Autodesk Fusion 360 part; units mm, degrees
note: some values were not read from the file. Chosen so that the rebuilt part matches the saved one: which face or edge a step refers to.
(part 2 of 2)
  spline S171 degree 3 poles (-22.5654, 6.7875) (-22.5201, 6.8696) (-22.457, 6.9326) (-22.3762, 6.9767) knots 0 0 0 0 1 1 1 1
  spline S172 degree 3 poles (-22.3762, 6.9767) (-22.2941, 7.022) (-22.2081, 7.045) (-22.1187, 7.045) knots 0 0 0 0 1 1 1 1
extrude "Extrude5" add sketch "Sketch5" along normal blind 2 contours L4 S0 S1 L5 S2 S3 L6 S4 S5 L7 S6 S7 | S8 L8 L9 S9 S10 L10 S11 L11 S12 | L12 S13 S14 L13 L14 L15 S15 S16 L16 S17 L17 S18 | S19 L18 S20 S21 L19 S22 | S23 S24 S25 S26 S27 S28 S29 L20 L21 S30 S31 L22 L23 S32 S33 S34 | L24 S35 S36 L25 L26 S37 S38 L27 L28 S39 S40 | S41 S42 S43 S44 S45 S46 S47 S48 S49 S50 S51 S52 S53 S54 L29 | S55 S56 L33 S57 L34 S58 S59 L35 S60 S61 L36 S62 L37 S63 S64 L38 | S65 S66 S67 S68 S69 S70 S71 S72 S73 S74 S75 S76 | S89 S90 S91 S92 S93 S94 S95 S96 S97 S98 S99 S100 | S101 S102 S103 S104 S105 S106 S107 S108 S109 S110 S111 S112 | S125 S126 S127 S128 S129 S130 S131 S132 S133 S134 S135 S136 | S137 S138 S139 S140 S141 S142 S143 S144 S145 S146 S147 S148 | S161 S162 S163 S164 S165 S166 S167 S168 S169 S170 S171 S172
extrude "Extrude2" [suppressed]
sketch "Sketch3" plane through (0, 0, 0) normal (1, 0, 0) x (0, 1, 0)
  line L0 (-62.5649, -7.7043) -> (-61.5927, -7.7068)
  spline S0 degree 3 poles (-61.5927, -7.7068) (-61.2707, -7.7117) (-61.1085, -7.8721) (-61.1066, -8.188) knots 0 0 0 0 1 1 1 1
  spline S1 degree 3 poles (-61.1066, -8.188) (-61.1085, -8.5155) (-61.2713, -8.6784) (-61.5952, -8.6765) knots 0 0 0 0 1 1 1 1
  line L1 (-61.5952, -8.6765) -> (-62.5625, -8.679)
  spline S2 degree 3 poles (-62.5625, -8.679) (-63.2089, -8.6741) (-63.5322, -8.9967) (-63.5322, -9.6462) knots 0 0 0 0 1 1 1 1
  spline S3 degree 3 poles (-63.5322, -9.6462) (-63.5322, -10.2915) (-63.2089, -10.6154) (-62.5625, -10.6184) knots 0 0 0 0 1 1 1 1
  line L2 (-62.5625, -10.6184) -> (-61.5952, -10.6184)
  spline S4 degree 3 poles (-61.5952, -10.6184) (-61.2713, -10.6252) (-61.1091, -10.7856) (-61.1091, -11.0996) knots 0 0 0 0 1 1 1 1
  spline S5 degree 3 poles (-61.1091, -11.0996) (-61.1091, -11.4241) (-61.2695, -11.5869) (-61.5903, -11.5882) knots 0 0 0 0 1 1 1 1
  line L3 (-61.5903, -11.5882) -> (-62.5625, -11.5882)
  spline S6 degree 3 poles (-62.5625, -11.5882) (-63.8573, -11.5882) (-64.5056, -10.9404) (-64.5068, -9.6438) knots 0 0 0 0 1 1 1 1
  spline S7 degree 3 poles (-64.5068, -9.6438) (-64.5068, -8.3496) (-63.8597, -7.7031) (-62.5649, -7.7043) knots 0 0 0 0 1 1 1 1
  spline S8 degree 3 poles (-60.1369, -7.6994) (-59.8112, -7.708) (-59.6471, -7.8666) (-59.6434, -8.1756) knots 0 0 0 0 1 1 1 1
  line L4 (-59.6434, -8.1756) -> (-59.6483, -10.6135)
  line L5 (-59.6483, -10.6135) -> (-57.7187, -10.6135)
  spline S9 degree 3 poles (-57.7187, -10.6135) (-57.3918, -10.6154) (-57.2277, -10.7788) (-57.2277, -11.1045) knots 0 0 0 0 1 1 1 1
  spline S10 degree 3 poles (-57.2277, -11.1045) (-57.2296, -11.4241) (-57.3899, -11.5851) (-57.7089, -11.5882) knots 0 0 0 0 1 1 1 1
  line L6 (-57.7089, -11.5882) -> (-60.1369, -11.5882)
  spline S11 degree 3 poles (-60.1369, -11.5882) (-60.4595, -11.5882) (-60.6217, -11.4315) (-60.623, -11.1169) knots 0 0 0 0 1 1 1 1
  line L7 (-60.623, -11.1169) -> (-60.623, -8.1904)
  spline S12 degree 3 poles (-60.623, -8.1904) (-60.6217, -7.8697) (-60.4595, -7.7062) (-60.1369, -7.6994) knots 0 0 0 0 1 1 1 1
  line L8 (-56.253, -7.6994) -> (-53.7954, -7.7043)
  spline S13 degree 3 poles (-53.7954, -7.7043) (-53.4931, -7.7093) (-53.3408, -7.8666) (-53.3389, -8.1756) knots 0 0 0 0 1 1 1 1
  spline S14 degree 3 poles (-53.3389, -8.1756) (-53.3389, -8.5063) (-53.503, -8.6741) (-53.8299, -8.679) knots 0 0 0 0 1 1 1 1
  line L9 (-53.8299, -8.679) -> (-55.7644, -8.679)
  line L10 (-55.7644, -8.679) -> (-55.7644, -10.6135)
  line L11 (-55.7644, -10.6135) -> (-53.8349, -10.6135)
  spline S15 degree 3 poles (-53.8349, -10.6135) (-53.5079, -10.6154) (-53.3438, -10.7788) (-53.3438, -11.1045) knots 0 0 0 0 1 1 1 1
  spline S16 degree 3 poles (-53.3438, -11.1045) (-53.3457, -11.4241) (-53.5061, -11.5851) (-53.825, -11.5882) knots 0 0 0 0 1 1 1 1
  line L12 (-53.825, -11.5882) -> (-56.253, -11.5882)
  spline S17 degree 3 poles (-56.253, -11.5882) (-56.5756, -11.5882) (-56.7379, -11.4315) (-56.7391, -11.1169) knots 0 0 0 0 1 1 1 1
  line L13 (-56.7391, -11.1169) -> (-56.7391, -8.1904)
  spline S18 degree 3 poles (-56.7391, -8.1904) (-56.7379, -7.8697) (-56.5756, -7.7062) (-56.253, -7.6994) knots 0 0 0 0 1 1 1 1
  spline S19 degree 3 poles (-55.5325, -9.6561) (-55.5294, -9.3341) (-55.369, -9.17) (-55.0513, -9.1651) knots 0 0 0 0 1 1 1 1
  line L14 (-55.0513, -9.1651) -> (-54.0742, -9.1651)
  spline S20 degree 3 poles (-54.0742, -9.1651) (-53.7504, -9.1688) (-53.5857, -9.3304) (-53.5807, -9.6512) knots 0 0 0 0 1 1 1 1
  spline S21 degree 3 poles (-53.5807, -9.6512) (-53.5875, -9.9757) (-53.751, -10.1373) (-54.0718, -10.1373) knots 0 0 0 0 1 1 1 1
  line L15 (-54.0718, -10.1373) -> (-55.0489, -10.1373)
  spline S22 degree 3 poles (-55.0489, -10.1373) (-55.3696, -10.1391) (-55.5313, -9.9787) (-55.5325, -9.6561) knots 0 0 0 0 1 1 1 1
  spline S23 degree 3 poles (-52.3617, -7.6945) (-52.2007, -7.6945) (-52.0792, -7.7352) (-51.9966, -7.8154) knots 0 0 0 0 1 1 1 1
  spline S24 degree 3 poles (-51.9966, -7.8154) (-51.9145, -7.8943) (-51.6264, -8.2324) (-51.1329, -8.8295) knots 0 0 0 0 1 1 1 1
  spline S25 degree 3 poles (-51.1329, -8.8295) (-50.6314, -8.2225) (-50.3396, -7.8795) (-50.257, -7.8006) knots 0 0 0 0 1 1 1 1
  spline S26 degree 3 poles (-50.257, -7.8006) (-50.1749, -7.7216) (-50.0534, -7.6821) (-49.8918, -7.6821) knots 0 0 0 0 1 1 1 1
  spline S27 degree 3 poles (-49.8918, -7.6821) (-49.7339, -7.6821) (-49.6123, -7.7235) (-49.5266, -7.8055) knots 0 0 0 0 1 1 1 1
  spline S28 degree 3 poles (-49.5266, -7.8055) (-49.4415, -7.8882) (-49.4008, -8.0103) (-49.4057, -8.1732) knots 0 0 0 0 1 1 1 1
  spline S29 degree 3 poles (-49.4057, -8.1732) (-49.4057, -8.3446) (-49.4914, -8.505) (-49.6623, -8.6543) knots 0 0 0 0 1 1 1 1
  line L16 (-49.6623, -8.6543) -> (-50.6567, -9.814)
  line L17 (-50.6567, -9.814) -> (-50.6592, -11.1045)
  spline S30 degree 3 poles (-50.6592, -11.1045) (-50.666, -11.4222) (-50.8288, -11.5832) (-51.1477, -11.5882) knots 0 0 0 0 1 1 1 1
  spline S31 degree 3 poles (-51.1477, -11.5882) (-51.4685, -11.5962) (-51.6289, -11.4302) (-51.6289, -11.0897) knots 0 0 0 0 1 1 1 1
  line L18 (-51.6289, -11.0897) -> (-51.6338, -9.8091)
  line L19 (-51.6338, -9.8091) -> (-52.5912, -8.6691)
  spline S32 degree 3 poles (-52.5912, -8.6691) (-52.7627, -8.518) (-52.8478, -8.357) (-52.8478, -8.1855) knots 0 0 0 0 1 1 1 1
  spline S33 degree 3 poles (-52.8478, -8.1855) (-52.8528, -8.0214) (-52.8133, -7.8986) (-52.7294, -7.8178) knots 0 0 0 0 1 1 1 1
  spline S34 degree 3 poles (-52.7294, -7.8178) (-52.6443, -7.7358) (-52.5215, -7.6945) (-52.3617, -7.6945) knots 0 0 0 0 1 1 1 1
  line L20 (-48.4804, -7.6994) -> (-46.0228, -7.7043)
  spline S35 degree 3 poles (-46.0228, -7.7043) (-45.7205, -7.7093) (-45.5682, -7.8666) (-45.5663, -8.1756) knots 0 0 0 0 1 1 1 1
  spline S36 degree 3 poles (-45.5663, -8.1756) (-45.5663, -8.5063) (-45.7304, -8.6741) (-46.0574, -8.679) knots 0 0 0 0 1 1 1 1
  line L21 (-46.0574, -8.679) -> (-46.7828, -8.679)
  line L22 (-46.7828, -8.679) -> (-46.7803, -11.1045)
  spline S37 degree 3 poles (-46.7803, -11.1045) (-46.784, -11.4241) (-46.9469, -11.5851) (-47.2689, -11.5882) knots 0 0 0 0 1 1 1 1
  spline S38 degree 3 poles (-47.2689, -11.5882) (-47.5934, -11.5882) (-47.755, -11.4315) (-47.755, -11.1169) knots 0 0 0 0 1 1 1 1
  line L23 (-47.755, -11.1169) -> (-47.7525, -8.679)
  line L24 (-47.7525, -8.679) -> (-48.4804, -8.679)
  spline S39 degree 3 poles (-48.4804, -8.679) (-48.8049, -8.679) (-48.9665, -8.5161) (-48.9665, -8.1904) knots 0 0 0 0 1 1 1 1
  spline S40 degree 3 poles (-48.9665, -8.1904) (-48.9653, -7.8697) (-48.803, -7.7062) (-48.4804, -7.6994) knots 0 0 0 0 1 1 1 1
  spline S41 degree 3 poles (-44.5941, -11.5906) (-44.6768, -11.5906) (-44.7563, -11.5703) (-44.8334, -11.5289) knots 0 0 0 0 1 1 1 1
  spline S42 degree 3 poles (-44.8334, -11.5289) (-44.9112, -11.4882) (-44.9716, -11.429) (-45.016, -11.3513) knots 0 0 0 0 1 1 1 1
  spline S43 degree 3 poles (-45.016, -11.3513) (-45.0592, -11.2723) (-45.0802, -11.1903) (-45.0802, -11.1045) knots 0 0 0 0 1 1 1 1
  spline S44 degree 3 poles (-45.0802, -11.1045) (-45.0802, -11.0206) (-44.8384, -10.4926) (-44.3547, -9.5204) knots 0 0 0 0 1 1 1 1
  spline S45 degree 3 poles (-44.3547, -9.5204) (-43.8699, -8.547) (-43.6065, -8.0214) (-43.5652, -7.9437) knots 0 0 0 0 1 1 1 1
  spline S46 degree 3 poles (-43.5652, -7.9437) (-43.5226, -7.8666) (-43.4628, -7.8067) (-43.385, -7.7636) knots 0 0 0 0 1 1 1 1
  spline S47 degree 3 poles (-43.385, -7.7636) (-43.3079, -7.721) (-43.2265, -7.6994) (-43.1407, -7.6994) knots 0 0 0 0 1 1 1 1
  spline S48 degree 3 poles (-43.1407, -7.6994) (-43.0569, -7.6994) (-42.9773, -7.721) (-42.9014, -7.7636) knots 0 0 0 0 1 1 1 1
  spline S49 degree 3 poles (-42.9014, -7.7636) (-42.8243, -7.8067) (-42.7645, -7.8666) (-42.7213, -7.9437) knots 0 0 0 0 1 1 1 1
  spline S50 degree 3 poles (-42.7213, -7.9437) (-42.6787, -8.0214) (-42.4141, -8.547) (-41.9267, -9.5204) knots 0 0 0 0 1 1 1 1
  spline S51 degree 3 poles (-41.9267, -9.5204) (-41.44, -10.4926) (-41.1964, -11.0206) (-41.1964, -11.1045) knots 0 0 0 0 1 1 1 1
  spline S52 degree 3 poles (-41.1964, -11.1045) (-41.1964, -11.1903) (-41.2186, -11.2723) (-41.263, -11.3513) knots 0 0 0 0 1 1 1 1
  spline S53 degree 3 poles (-41.263, -11.3513) (-41.3062, -11.429) (-41.3666, -11.4882) (-41.4456, -11.5289) knots 0 0 0 0 1 1 1 1
  spline S54 degree 3 poles (-41.4456, -11.5289) (-41.5233, -11.5703) (-41.6023, -11.5906) (-41.6825, -11.5906) knots 0 0 0 0 1 1 1 1
  line L25 (-41.6825, -11.5906) -> (-44.5941, -11.5906)
  line L26 (-42.477, -10.611) -> (-43.1407, -9.244)
  line L27 (-43.1407, -9.244) -> (-43.8094, -10.611)
  line L28 (-43.8094, -10.611) -> (-42.477, -10.611)
  spline S55 degree 3 poles (-36.5839, -7.7043) (-35.4507, -7.7031) (-34.8832, -8.3502) (-34.8814, -9.6462) knots 0 0 0 0 1 1 1 1
  spline S56 degree 3 poles (-34.8814, -9.6462) (-34.8801, -9.9707) (-35.0418, -10.1317) (-35.3675, -10.1299) knots 0 0 0 0 1 1 1 1
  line L29 (-35.3675, -10.1299) -> (-37.3118, -10.1274)
  spline S57 degree 3 poles (-37.3118, -10.1274) (-37.3088, -10.4531) (-37.0669, -10.6172) (-36.5864, -10.6184) knots 0 0 0 0 1 1 1 1
  line L30 (-36.5864, -10.6184) -> (-35.365, -10.6135)
  spline S58 degree 3 poles (-35.365, -10.6135) (-35.0479, -10.6154) (-34.8863, -10.7782) (-34.8814, -11.1021) knots 0 0 0 0 1 1 1 1
  spline S59 degree 3 poles (-34.8814, -11.1021) (-34.8832, -11.4278) (-35.0455, -11.5894) (-35.3675, -11.5882) knots 0 0 0 0 1 1 1 1
  line L31 (-35.3675, -11.5882) -> (-36.579, -11.5882)
  spline S60 degree 3 poles (-36.579, -11.5882) (-37.7159, -11.5869) (-38.2853, -10.9386) (-38.2865, -9.6438) knots 0 0 0 0 1 1 1 1
  spline S61 degree 3 poles (-38.2865, -9.6438) (-38.2853, -9.323) (-38.123, -9.162) (-37.8004, -9.1602) knots 0 0 0 0 1 1 1 1
  line L32 (-37.8004, -9.1602) -> (-35.856, -9.1626)
  spline S62 degree 3 poles (-35.856, -9.1626) (-35.856, -8.8388) (-36.0954, -8.6778) (-36.5741, -8.679) knots 0 0 0 0 1 1 1 1
  line L33 (-36.5741, -8.679) -> (-37.7955, -8.679)
  spline S63 degree 3 poles (-37.7955, -8.679) (-38.1162, -8.671) (-38.2803, -8.5075) (-38.2865, -8.188) knots 0 0 0 0 1 1 1 1
  spline S64 degree 3 poles (-38.2865, -8.188) (-38.2785, -7.8641) (-38.115, -7.7031) (-37.7955, -7.7043) knots 0 0 0 0 1 1 1 1
  line L34 (-37.7955, -7.7043) -> (-36.5839, -7.7043)
  spline S65 degree 3 poles (-32.4583, -7.7043) (-32.1326, -7.7043) (-31.8155, -7.7882) (-31.5058, -7.956) knots 0 0 0 0 1 1 1 1
  spline S66 degree 3 poles (-31.5058, -7.956) (-31.1949, -8.1238) (-30.9519, -8.3644) (-30.7755, -8.6765) knots 0 0 0 0 1 1 1 1
  spline S67 degree 3 poles (-30.7755, -8.6765) (-30.5997, -8.9874) (-30.5115, -9.3119) (-30.5115, -9.6487) knots 0 0 0 0 1 1 1 1
  spline S68 degree 3 poles (-30.5115, -9.6487) (-30.5115, -9.9861) (-30.5972, -10.3094) (-30.7681, -10.6184) knots 0 0 0 0 1 1 1 1
  spline S69 degree 3 poles (-30.7681, -10.6184) (-30.9396, -10.9263) (-31.1795, -11.1656) (-31.4886, -11.3365) knots 0 0 0 0 1 1 1 1
  spline S70 degree 3 poles (-31.4886, -11.3365) (-31.7982, -11.508) (-32.1215, -11.5931) (-32.4583, -11.5931) knots 0 0 0 0 1 1 1 1
  spline S71 degree 3 poles (-32.4583, -11.5931) (-32.7939, -11.5931) (-33.1165, -11.508) (-33.4256, -11.3365) knots 0 0 0 0 1 1 1 1
  spline S72 degree 3 poles (-33.4256, -11.3365) (-33.7352, -11.1656) (-33.9752, -10.9263) (-34.1461, -10.6184) knots 0 0 0 0 1 1 1 1
  spline S73 degree 3 poles (-34.1461, -10.6184) (-34.3176, -10.3094) (-34.4027, -9.9861) (-34.4027, -9.6487) knots 0 0 0 0 1 1 1 1
  spline S74 degree 3 poles (-34.4027, -9.6487) (-34.4027, -9.3119) (-34.3163, -8.9874) (-34.1436, -8.6765) knots 0 0 0 0 1 1 1 1
  spline S75 degree 3 poles (-34.1436, -8.6765) (-33.9696, -8.3644) (-33.7278, -8.1238) (-33.4182, -7.956) knots 0 0 0 0 1 1 1 1
  spline S76 degree 3 poles (-33.4182, -7.956) (-33.1072, -7.7882) (-32.7877, -7.7043) (-32.4583, -7.7043) knots 0 0 0 0 1 1 1 1
  spline S77 degree 3 poles (-32.4558, -8.6716) (-32.6205, -8.6716) (-32.7803, -8.7135) (-32.9345, -8.7974) knots 0 0 0 0 1 1 1 1
  spline S78 degree 3 poles (-32.9345, -8.7974) (-33.0894, -8.8801) (-33.2103, -8.9991) (-33.2972, -9.1552) knots 0 0 0 0 1 1 1 1
  spline S79 degree 3 poles (-33.2972, -9.1552) (-33.3848, -9.3119) (-33.428, -9.4748) (-33.428, -9.6438) knots 0 0 0 0 1 1 1 1
  spline S80 degree 3 poles (-33.428, -9.6438) (-33.428, -9.8134) (-33.3855, -9.9757) (-33.2997, -10.1299) knots 0 0 0 0 1 1 1 1
  spline S81 degree 3 poles (-33.2997, -10.1299) (-33.2146, -10.2829) (-33.0943, -10.4025) (-32.9395, -10.4877) knots 0 0 0 0 1 1 1 1
  spline S82 degree 3 poles (-32.9395, -10.4877) (-32.7852, -10.5734) (-32.6236, -10.616) (-32.4558, -10.616) knots 0 0 0 0 1 1 1 1
  spline S83 degree 3 poles (-32.4558, -10.616) (-32.2868, -10.616) (-32.1246, -10.5734) (-31.9697, -10.4877) knots 0 0 0 0 1 1 1 1
  spline S84 degree 3 poles (-31.9697, -10.4877) (-31.8155, -10.4025) (-31.6952, -10.2829) (-31.6095, -10.1299) knots 0 0 0 0 1 1 1 1
  spline S85 degree 3 poles (-31.6095, -10.1299) (-31.5244, -9.9757) (-31.4812, -9.8134) (-31.4812, -9.6438) knots 0 0 0 0 1 1 1 1
  spline S86 degree 3 poles (-31.4812, -9.6438) (-31.4812, -9.4748) (-31.525, -9.3119) (-31.612, -9.1552) knots 0 0 0 0 1 1 1 1
  spline S87 degree 3 poles (-31.612, -9.1552) (-31.6995, -8.9991) (-31.8211, -8.8801) (-31.9771, -8.7974) knots 0 0 0 0 1 1 1 1
  spline S88 degree 3 poles (-31.9771, -8.7974) (-32.132, -8.7135) (-32.2917, -8.6716) (-32.4558, -8.6716) knots 0 0 0 0 1 1 1 1
  spline S89 degree 3 poles (-32.4583, -9.17) (-32.3781, -9.17) (-32.2998, -9.1916) (-32.2239, -9.2342) knots 0 0 0 0 1 1 1 1
  spline S90 degree 3 poles (-32.2239, -9.2342) (-32.1468, -9.2755) (-32.0869, -9.3347) (-32.0438, -9.4118) knots 0 0 0 0 1 1 1 1
  spline S91 degree 3 poles (-32.0438, -9.4118) (-31.9993, -9.4877) (-31.9771, -9.5685) (-31.9771, -9.6536) knots 0 0 0 0 1 1 1 1
  spline S92 degree 3 poles (-31.9771, -9.6536) (-31.9771, -9.7375) (-31.9987, -9.8184) (-32.0413, -9.8955) knots 0 0 0 0 1 1 1 1
  spline S93 degree 3 poles (-32.0413, -9.8955) (-32.0845, -9.9713) (-32.1437, -10.0306) (-32.219, -10.0731) knots 0 0 0 0 1 1 1 1
  spline S94 degree 3 poles (-32.219, -10.0731) (-32.2948, -10.1145) (-32.3744, -10.1348) (-32.4583, -10.1348) knots 0 0 0 0 1 1 1 1
  spline S95 degree 3 poles (-32.4583, -10.1348) (-32.544, -10.1348) (-32.6255, -10.1145) (-32.7026, -10.0731) knots 0 0 0 0 1 1 1 1
  spline S96 degree 3 poles (-32.7026, -10.0731) (-32.7785, -10.0306) (-32.8377, -9.9713) (-32.8802, -9.8955) knots 0 0 0 0 1 1 1 1
  spline S97 degree 3 poles (-32.8802, -9.8955) (-32.9216, -9.8184) (-32.9419, -9.7375) (-32.9419, -9.6536) knots 0 0 0 0 1 1 1 1
  spline S98 degree 3 poles (-32.9419, -9.6536) (-32.9419, -9.5685) (-32.921, -9.4877) (-32.8778, -9.4118) knots 0 0 0 0 1 1 1 1
  spline S99 degree 3 poles (-32.8778, -9.4118) (-32.8352, -9.3347) (-32.776, -9.2755) (-32.7001, -9.2342) knots 0 0 0 0 1 1 1 1
  spline S100 degree 3 poles (-32.7001, -9.2342) (-32.623, -9.1916) (-32.5422, -9.17) (-32.4583, -9.17) knots 0 0 0 0 1 1 1 1
  spline S101 degree 3 poles (-28.0838, -7.7043) (-27.7581, -7.7043) (-27.441, -7.7882) (-27.1313, -7.956) knots 0 0 0 0 1 1 1 1
  spline S102 degree 3 poles (-27.1313, -7.956) (-26.8204, -8.1238) (-26.5774, -8.3644) (-26.401, -8.6765) knots 0 0 0 0 1 1 1 1
  spline S103 degree 3 poles (-26.401, -8.6765) (-26.2252, -8.9874) (-26.1369, -9.3119) (-26.1369, -9.6487) knots 0 0 0 0 1 1 1 1
  spline S104 degree 3 poles (-26.1369, -9.6487) (-26.1369, -9.9861) (-26.2227, -10.3094) (-26.3936, -10.6184) knots 0 0 0 0 1 1 1 1
  spline S105 degree 3 poles (-26.3936, -10.6184) (-26.5651, -10.9263) (-26.805, -11.1656) (-27.1141, -11.3365) knots 0 0 0 0 1 1 1 1
  spline S106 degree 3 poles (-27.1141, -11.3365) (-27.4237, -11.508) (-27.747, -11.5931) (-28.0838, -11.5931) knots 0 0 0 0 1 1 1 1
  spline S107 degree 3 poles (-28.0838, -11.5931) (-28.4194, -11.5931) (-28.742, -11.508) (-29.051, -11.3365) knots 0 0 0 0 1 1 1 1
  spline S108 degree 3 poles (-29.051, -11.3365) (-29.3607, -11.1656) (-29.6007, -10.9263) (-29.7716, -10.6184) knots 0 0 0 0 1 1 1 1
  spline S109 degree 3 poles (-29.7716, -10.6184) (-29.943, -10.3094) (-30.0282, -9.9861) (-30.0282, -9.6487) knots 0 0 0 0 1 1 1 1
  spline S110 degree 3 poles (-30.0282, -9.6487) (-30.0282, -9.3119) (-29.9418, -8.9874) (-29.7691, -8.6765) knots 0 0 0 0 1 1 1 1
  spline S111 degree 3 poles (-29.7691, -8.6765) (-29.5951, -8.3644) (-29.3533, -8.1238) (-29.0436, -7.956) knots 0 0 0 0 1 1 1 1
  spline S112 degree 3 poles (-29.0436, -7.956) (-28.7327, -7.7882) (-28.4132, -7.7043) (-28.0838, -7.7043) knots 0 0 0 0 1 1 1 1
  spline S113 degree 3 poles (-28.0813, -8.6716) (-28.246, -8.6716) (-28.4058, -8.7135) (-28.56, -8.7974) knots 0 0 0 0 1 1 1 1
  spline S114 degree 3 poles (-28.56, -8.7974) (-28.7149, -8.8801) (-28.8358, -8.9991) (-28.9227, -9.1552) knots 0 0 0 0 1 1 1 1
  spline S115 degree 3 poles (-28.9227, -9.1552) (-29.0103, -9.3119) (-29.0535, -9.4748) (-29.0535, -9.6438) knots 0 0 0 0 1 1 1 1
  spline S116 degree 3 poles (-29.0535, -9.6438) (-29.0535, -9.8134) (-29.0109, -9.9757) (-28.9252, -10.1299) knots 0 0 0 0 1 1 1 1
  spline S117 degree 3 poles (-28.9252, -10.1299) (-28.8401, -10.2829) (-28.7198, -10.4025) (-28.565, -10.4877) knots 0 0 0 0 1 1 1 1
  spline S118 degree 3 poles (-28.565, -10.4877) (-28.4107, -10.5734) (-28.2491, -10.616) (-28.0813, -10.616) knots 0 0 0 0 1 1 1 1
  spline S119 degree 3 poles (-28.0813, -10.616) (-27.9123, -10.616) (-27.7501, -10.5734) (-27.5952, -10.4877) knots 0 0 0 0 1 1 1 1
  spline S120 degree 3 poles (-27.5952, -10.4877) (-27.441, -10.4025) (-27.3207, -10.2829) (-27.235, -10.1299) knots 0 0 0 0 1 1 1 1
  spline S121 degree 3 poles (-27.235, -10.1299) (-27.1498, -9.9757) (-27.1067, -9.8134) (-27.1067, -9.6438) knots 0 0 0 0 1 1 1 1
  spline S122 degree 3 poles (-27.1067, -9.6438) (-27.1067, -9.4748) (-27.1505, -9.3119) (-27.2374, -9.1552) knots 0 0 0 0 1 1 1 1
  spline S123 degree 3 poles (-27.2374, -9.1552) (-27.325, -8.9991) (-27.4466, -8.8801) (-27.6026, -8.7974) knots 0 0 0 0 1 1 1 1
  spline S124 degree 3 poles (-27.6026, -8.7974) (-27.7575, -8.7135) (-27.9172, -8.6716) (-28.0813, -8.6716) knots 0 0 0 0 1 1 1 1
  spline S125 degree 3 poles (-28.0838, -9.17) (-28.0036, -9.17) (-27.9253, -9.1916) (-27.8494, -9.2342) knots 0 0 0 0 1 1 1 1
  spline S126 degree 3 poles (-27.8494, -9.2342) (-27.7723, -9.2755) (-27.7124, -9.3347) (-27.6693, -9.4118) knots 0 0 0 0 1 1 1 1
  spline S127 degree 3 poles (-27.6693, -9.4118) (-27.6248, -9.4877) (-27.6026, -9.5685) (-27.6026, -9.6536) knots 0 0 0 0 1 1 1 1
  spline S128 degree 3 poles (-27.6026, -9.6536) (-27.6026, -9.7375) (-27.6242, -9.8184) (-27.6668, -9.8955) knots 0 0 0 0 1 1 1 1
  spline S129 degree 3 poles (-27.6668, -9.8955) (-27.71, -9.9713) (-27.7692, -10.0306) (-27.8444, -10.0731) knots 0 0 0 0 1 1 1 1
  spline S130 degree 3 poles (-27.8444, -10.0731) (-27.9203, -10.1145) (-27.9999, -10.1348) (-28.0838, -10.1348) knots 0 0 0 0 1 1 1 1
  spline S131 degree 3 poles (-28.0838, -10.1348) (-28.1695, -10.1348) (-28.251, -10.1145) (-28.3281, -10.0731) knots 0 0 0 0 1 1 1 1
  spline S132 degree 3 poles (-28.3281, -10.0731) (-28.4039, -10.0306) (-28.4632, -9.9713) (-28.5057, -9.8955) knots 0 0 0 0 1 1 1 1
  spline S133 degree 3 poles (-28.5057, -9.8955) (-28.5471, -9.8184) (-28.5674, -9.7375) (-28.5674, -9.6536) knots 0 0 0 0 1 1 1 1
  spline S134 degree 3 poles (-28.5674, -9.6536) (-28.5674, -9.5685) (-28.5464, -9.4877) (-28.5033, -9.4118) knots 0 0 0 0 1 1 1 1
  spline S135 degree 3 poles (-28.5033, -9.4118) (-28.4607, -9.3347) (-28.4015, -9.2755) (-28.3256, -9.2342) knots 0 0 0 0 1 1 1 1
  spline S136 degree 3 poles (-28.3256, -9.2342) (-28.2485, -9.1916) (-28.1677, -9.17) (-28.0838, -9.17) knots 0 0 0 0 1 1 1 1
  spline S137 degree 3 poles (-23.7093, -7.7043) (-23.3836, -7.7043) (-23.0665, -7.7882) (-22.7568, -7.956) knots 0 0 0 0 1 1 1 1
  spline S138 degree 3 poles (-22.7568, -7.956) (-22.4459, -8.1238) (-22.2029, -8.3644) (-22.0265, -8.6765) knots 0 0 0 0 1 1 1 1
  spline S139 degree 3 poles (-22.0265, -8.6765) (-21.8506, -8.9874) (-21.7624, -9.3119) (-21.7624, -9.6487) knots 0 0 0 0 1 1 1 1
  spline S140 degree 3 poles (-21.7624, -9.6487) (-21.7624, -9.9861) (-21.8482, -10.3094) (-22.0191, -10.6184) knots 0 0 0 0 1 1 1 1
  spline S141 degree 3 poles (-22.0191, -10.6184) (-22.1905, -10.9263) (-22.4305, -11.1656) (-22.7396, -11.3365) knots 0 0 0 0 1 1 1 1
  spline S142 degree 3 poles (-22.7396, -11.3365) (-23.0492, -11.508) (-23.3725, -11.5931) (-23.7093, -11.5931) knots 0 0 0 0 1 1 1 1
  spline S143 degree 3 poles (-23.7093, -11.5931) (-24.0449, -11.5931) (-24.3675, -11.508) (-24.6765, -11.3365) knots 0 0 0 0 1 1 1 1
  spline S144 degree 3 poles (-24.6765, -11.3365) (-24.9862, -11.1656) (-25.2262, -10.9263) (-25.397, -10.6184) knots 0 0 0 0 1 1 1 1
  spline S145 degree 3 poles (-25.397, -10.6184) (-25.5685, -10.3094) (-25.6537, -9.9861) (-25.6537, -9.6487) knots 0 0 0 0 1 1 1 1
  spline S146 degree 3 poles (-25.6537, -9.6487) (-25.6537, -9.3119) (-25.5673, -8.9874) (-25.3946, -8.6765) knots 0 0 0 0 1 1 1 1
  spline S147 degree 3 poles (-25.3946, -8.6765) (-25.2206, -8.3644) (-24.9788, -8.1238) (-24.6691, -7.956) knots 0 0 0 0 1 1 1 1
  spline S148 degree 3 poles (-24.6691, -7.956) (-24.3582, -7.7882) (-24.0387, -7.7043) (-23.7093, -7.7043) knots 0 0 0 0 1 1 1 1
  spline S149 degree 3 poles (-23.7068, -8.6716) (-23.8715, -8.6716) (-24.0313, -8.7135) (-24.1855, -8.7974) knots 0 0 0 0 1 1 1 1
  spline S150 degree 3 poles (-24.1855, -8.7974) (-24.3403, -8.8801) (-24.4613, -8.9991) (-24.5482, -9.1552) knots 0 0 0 0 1 1 1 1
  spline S151 degree 3 poles (-24.5482, -9.1552) (-24.6358, -9.3119) (-24.679, -9.4748) (-24.679, -9.6438) knots 0 0 0 0 1 1 1 1
  spline S152 degree 3 poles (-24.679, -9.6438) (-24.679, -9.8134) (-24.6364, -9.9757) (-24.5507, -10.1299) knots 0 0 0 0 1 1 1 1
  spline S153 degree 3 poles (-24.5507, -10.1299) (-24.4656, -10.2829) (-24.3453, -10.4025) (-24.1904, -10.4877) knots 0 0 0 0 1 1 1 1
  spline S154 degree 3 poles (-24.1904, -10.4877) (-24.0362, -10.5734) (-23.8746, -10.616) (-23.7068, -10.616) knots 0 0 0 0 1 1 1 1
  spline S155 degree 3 poles (-23.7068, -10.616) (-23.5378, -10.616) (-23.3756, -10.5734) (-23.2207, -10.4877) knots 0 0 0 0 1 1 1 1
  spline S156 degree 3 poles (-23.2207, -10.4877) (-23.0665, -10.4025) (-22.9462, -10.2829) (-22.8605, -10.1299) knots 0 0 0 0 1 1 1 1
  spline S157 degree 3 poles (-22.8605, -10.1299) (-22.7753, -9.9757) (-22.7322, -9.8134) (-22.7322, -9.6438) knots 0 0 0 0 1 1 1 1
  spline S158 degree 3 poles (-22.7322, -9.6438) (-22.7322, -9.4748) (-22.776, -9.3119) (-22.8629, -9.1552) knots 0 0 0 0 1 1 1 1
  spline S159 degree 3 poles (-22.8629, -9.1552) (-22.9505, -8.9991) (-23.0721, -8.8801) (-23.2281, -8.7974) knots 0 0 0 0 1 1 1 1
  spline S160 degree 3 poles (-23.2281, -8.7974) (-23.383, -8.7135) (-23.5427, -8.6716) (-23.7068, -8.6716) knots 0 0 0 0 1 1 1 1
  spline S161 degree 3 poles (-23.7093, -9.17) (-23.6291, -9.17) (-23.5507, -9.1916) (-23.4749, -9.2342) knots 0 0 0 0 1 1 1 1
  spline S162 degree 3 poles (-23.4749, -9.2342) (-23.3978, -9.2755) (-23.3379, -9.3347) (-23.2947, -9.4118) knots 0 0 0 0 1 1 1 1
  spline S163 degree 3 poles (-23.2947, -9.4118) (-23.2503, -9.4877) (-23.2281, -9.5685) (-23.2281, -9.6536) knots 0 0 0 0 1 1 1 1
  spline S164 degree 3 poles (-23.2281, -9.6536) (-23.2281, -9.7375) (-23.2497, -9.8184) (-23.2923, -9.8955) knots 0 0 0 0 1 1 1 1
  spline S165 degree 3 poles (-23.2923, -9.8955) (-23.3355, -9.9713) (-23.3947, -10.0306) (-23.4699, -10.0731) knots 0 0 0 0 1 1 1 1
  spline S166 degree 3 poles (-23.4699, -10.0731) (-23.5458, -10.1145) (-23.6254, -10.1348) (-23.7093, -10.1348) knots 0 0 0 0 1 1 1 1
  spline S167 degree 3 poles (-23.7093, -10.1348) (-23.795, -10.1348) (-23.8765, -10.1145) (-23.9536, -10.0731) knots 0 0 0 0 1 1 1 1
  spline S168 degree 3 poles (-23.9536, -10.0731) (-24.0294, -10.0306) (-24.0887, -9.9713) (-24.1312, -9.8955) knots 0 0 0 0 1 1 1 1
  spline S169 degree 3 poles (-24.1312, -9.8955) (-24.1726, -9.8184) (-24.1929, -9.7375) (-24.1929, -9.6536) knots 0 0 0 0 1 1 1 1
  spline S170 degree 3 poles (-24.1929, -9.6536) (-24.1929, -9.5685) (-24.1719, -9.4877) (-24.1288, -9.4118) knots 0 0 0 0 1 1 1 1
  spline S171 degree 3 poles (-24.1288, -9.4118) (-24.0862, -9.3347) (-24.027, -9.2755) (-23.9511, -9.2342) knots 0 0 0 0 1 1 1 1
  spline S172 degree 3 poles (-23.9511, -9.2342) (-23.874, -9.1916) (-23.7932, -9.17) (-23.7093, -9.17) knots 0 0 0 0 1 1 1 1
sketch "Sketch4" plane through (5, 0, 0) normal (1, 0, 0) x (0, 1, 0)
  spline S0 degree 3 poles (-29.4282, 6.6218) (-29.4282, 6.9634) (-29.3407, 7.2924) (-29.1655, 7.6077) knots 0 0 0 0 1 1 1 1
  spline S1 degree 3 poles (-29.1655, 7.6077) (-28.9891, 7.9242) (-28.7439, 8.1682) (-28.4298, 8.3384) knots 0 0 0 0 1 1 1 1
  spline S2 degree 3 poles (-28.4298, 8.3384) (-28.1146, 8.5085) (-27.7905, 8.5936) (-27.4565, 8.5936) knots 0 0 0 0 1 1 1 1
  spline S3 degree 3 poles (-27.4565, 8.5936) (-27.1262, 8.5936) (-26.8046, 8.5085) (-26.4906, 8.3384) knots 0 0 0 0 1 1 1 1
  spline S4 degree 3 poles (-26.4906, 8.3384) (-26.1753, 8.1682) (-25.9288, 7.9242) (-25.7499, 7.6077) knots 0 0 0 0 1 1 1 1
  spline S5 degree 3 poles (-25.7499, 7.6077) (-25.5716, 7.2924) (-25.4822, 6.9634) (-25.4822, 6.6218) knots 0 0 0 0 1 1 1 1
  spline S6 degree 3 poles (-25.4822, 6.6218) (-25.4822, 6.2796) (-25.5691, 5.9518) (-25.7424, 5.6384) knots 0 0 0 0 1 1 1 1
  spline S7 degree 3 poles (-25.7424, 5.6384) (-25.9163, 5.3263) (-26.1597, 5.0835) (-26.4731, 4.9103) knots 0 0 0 0 1 1 1 1
  spline S8 degree 3 poles (-26.4731, 4.9103) (-26.7871, 4.7363) (-27.1149, 4.65) (-27.4565, 4.65) knots 0 0 0 0 1 1 1 1
  spline S9 degree 3 poles (-27.4565, 4.65) (-27.7968, 4.65) (-28.1239, 4.7363) (-28.4373, 4.9103) knots 0 0 0 0 1 1 1 1
  spline S10 degree 3 poles (-28.4373, 4.9103) (-28.7514, 5.0835) (-28.9947, 5.3263) (-29.168, 5.6384) knots 0 0 0 0 1 1 1 1
  spline S11 degree 3 poles (-29.168, 5.6384) (-29.3419, 5.9518) (-29.4282, 6.2796) (-29.4282, 6.6218) knots 0 0 0 0 1 1 1 1
  spline S12 degree 3 poles (-37.305, 7.6052) (-37.6303, 7.6133) (-37.7967, 7.7791) (-37.803, 8.1031) knots 0 0 0 0 1 1 1 1
  spline S13 degree 3 poles (-37.803, 8.1031) (-37.7948, 8.4316) (-37.629, 8.5948) (-37.305, 8.5936) knots 0 0 0 0 1 1 1 1
  line L0 (-37.305, 8.5936) -> (-36.0764, 8.5936)
  spline S14 degree 3 poles (-36.0764, 8.5936) (-34.9272, 8.5948) (-34.3517, 7.9386) (-34.3498, 6.6243) knots 0 0 0 0 1 1 1 1
  spline S15 degree 3 poles (-34.3498, 6.6243) (-34.3486, 6.2953) (-34.5125, 6.132) (-34.8428, 6.1339) knots 0 0 0 0 1 1 1 1
  line L1 (-34.8428, 6.1339) -> (-36.8146, 6.1364)
  spline S16 degree 3 poles (-36.8146, 6.1364) (-36.8114, 5.8061) (-36.5662, 5.6397) (-36.0789, 5.6384) knots 0 0 0 0 1 1 1 1
  line L2 (-36.0789, 5.6384) -> (-34.8403, 5.6434)
  spline S17 degree 3 poles (-34.8403, 5.6434) (-34.5187, 5.6415) (-34.3548, 5.4764) (-34.3498, 5.148) knots 0 0 0 0 1 1 1 1
  spline S18 degree 3 poles (-34.3498, 5.148) (-34.3517, 4.8177) (-34.5162, 4.6538) (-34.8428, 4.655) knots 0 0 0 0 1 1 1 1
  line L3 (-34.8428, 4.655) -> (-36.0714, 4.655)
  spline S19 degree 3 poles (-36.0714, 4.655) (-37.2243, 4.6563) (-37.8017, 5.3137) (-37.803, 6.6268) knots 0 0 0 0 1 1 1 1
  spline S20 degree 3 poles (-37.803, 6.6268) (-37.8017, 6.9521) (-37.6372, 7.1154) (-37.31, 7.1173) knots 0 0 0 0 1 1 1 1
  line L4 (-37.31, 7.1173) -> (-35.3382, 7.1147)
  spline S21 degree 3 poles (-35.3382, 7.1147) (-35.3382, 7.4432) (-35.5809, 7.6064) (-36.0664, 7.6052) knots 0 0 0 0 1 1 1 1
  line L5 (-36.0664, 7.6052) -> (-37.305, 7.6052)
  spline S22 degree 3 poles (-53.3127, 6.6193) (-53.3196, 6.2903) (-53.4854, 6.1264) (-53.8107, 6.1264) knots 0 0 0 0 1 1 1 1
  line L6 (-53.8107, 6.1264) -> (-54.8016, 6.1264)
  spline S23 degree 3 poles (-54.8016, 6.1264) (-55.1268, 6.1245) (-55.2907, 6.2871) (-55.292, 6.6143) knots 0 0 0 0 1 1 1 1
  spline S24 degree 3 poles (-55.292, 6.6143) (-55.2889, 6.9408) (-55.1262, 7.1072) (-54.8041, 7.1122) knots 0 0 0 0 1 1 1 1
  line L7 (-54.8041, 7.1122) -> (-53.8132, 7.1122)
  spline S25 degree 3 poles (-53.8132, 7.1122) (-53.4847, 7.1085) (-53.3177, 6.9446) (-53.3127, 6.6193) knots 0 0 0 0 1 1 1 1
  line L8 (-61.4351, 4.655) -> (-62.421, 4.655)
  spline S26 degree 3 poles (-62.421, 4.655) (-63.7341, 4.655) (-64.3915, 5.3119) (-64.3928, 6.6268) knots 0 0 0 0 1 1 1 1
  spline S27 degree 3 poles (-64.3928, 6.6268) (-64.3928, 7.9392) (-63.7366, 8.5948) (-62.4235, 8.5936) knots 0 0 0 0 1 1 1 1
  line L9 (-62.4235, 8.5936) -> (-61.4376, 8.5911)
  spline S28 degree 3 poles (-61.4376, 8.5911) (-61.1111, 8.5861) (-60.9466, 8.4234) (-60.9447, 8.1031) knots 0 0 0 0 1 1 1 1
  spline S29 degree 3 poles (-60.9447, 8.1031) (-60.9466, 7.771) (-61.1117, 7.6058) (-61.4401, 7.6077) knots 0 0 0 0 1 1 1 1
  line L10 (-61.4401, 7.6077) -> (-62.421, 7.6052)
  spline S30 degree 3 poles (-62.421, 7.6052) (-63.0766, 7.6102) (-63.4044, 7.283) (-63.4044, 6.6243) knots 0 0 0 0 1 1 1 1
  spline S31 degree 3 poles (-63.4044, 6.6243) (-63.4044, 5.97) (-63.0766, 5.6415) (-62.421, 5.6384) knots 0 0 0 0 1 1 1 1
  line L11 (-62.421, 5.6384) -> (-61.4401, 5.6384)
  spline S32 degree 3 poles (-61.4401, 5.6384) (-61.1117, 5.6315) (-60.9472, 5.4689) (-60.9472, 5.1505) knots 0 0 0 0 1 1 1 1
  spline S33 degree 3 poles (-60.9472, 5.1505) (-60.9472, 4.8214) (-61.1098, 4.6563) (-61.4351, 4.655) knots 0 0 0 0 1 1 1 1
  spline S34 degree 3 poles (-52.3093, 7.6152) (-52.4832, 7.7685) (-52.5695, 7.9317) (-52.5695, 8.1056) knots 0 0 0 0 1 1 1 1
  spline S35 degree 3 poles (-52.5695, 8.1056) (-52.5745, 8.272) (-52.5345, 8.3965) (-52.4494, 8.4785) knots 0 0 0 0 1 1 1 1
  spline S36 degree 3 poles (-52.4494, 8.4785) (-52.3631, 8.5617) (-52.2386, 8.6036) (-52.0766, 8.6036) knots 0 0 0 0 1 1 1 1
  spline S37 degree 3 poles (-52.0766, 8.6036) (-51.9133, 8.6036) (-51.79, 8.5623) (-51.7062, 8.481) knots 0 0 0 0 1 1 1 1
  spline S38 degree 3 poles (-51.7062, 8.481) (-51.623, 8.4009) (-51.3309, 8.0581) (-50.8304, 7.4526) knots 0 0 0 0 1 1 1 1
  spline S39 degree 3 poles (-50.8304, 7.4526) (-50.3218, 8.0681) (-50.026, 8.4159) (-49.9421, 8.496) knots 0 0 0 0 1 1 1 1
  spline S40 degree 3 poles (-49.9421, 8.496) (-49.8589, 8.5761) (-49.7357, 8.6161) (-49.5718, 8.6161) knots 0 0 0 0 1 1 1 1
  spline S41 degree 3 poles (-49.5718, 8.6161) (-49.4116, 8.6161) (-49.2884, 8.5742) (-49.2015, 8.491) knots 0 0 0 0 1 1 1 1
  spline S42 degree 3 poles (-49.2015, 8.491) (-49.1151, 8.4072) (-49.0738, 8.2833) (-49.0788, 8.1182) knots 0 0 0 0 1 1 1 1
  spline S43 degree 3 poles (-49.0788, 8.1182) (-49.0788, 7.9442) (-49.1658, 7.7816) (-49.3391, 7.6302) knots 0 0 0 0 1 1 1 1
  line L12 (-49.3391, 7.6302) -> (-50.3475, 6.4542)
  line L13 (-50.3475, 6.4542) -> (-50.35, 5.1455)
  spline S44 degree 3 poles (-50.35, 5.1455) (-50.3569, 4.8233) (-50.522, 4.66) (-50.8454, 4.655) knots 0 0 0 0 1 1 1 1
  spline S45 degree 3 poles (-50.8454, 4.655) (-51.1707, 4.6469) (-51.3334, 4.8152) (-51.3334, 5.1605) knots 0 0 0 0 1 1 1 1
  line L14 (-51.3334, 5.1605) -> (-51.3384, 6.4592)
  line L15 (-51.3384, 6.4592) -> (-52.3093, 7.6152)
  spline S46 degree 3 poles (-33.8644, 6.6218) (-33.8644, 6.9634) (-33.7768, 7.2924) (-33.6017, 7.6077) knots 0 0 0 0 1 1 1 1
  spline S47 degree 3 poles (-33.6017, 7.6077) (-33.4253, 7.9242) (-33.18, 8.1682) (-32.866, 8.3384) knots 0 0 0 0 1 1 1 1
  spline S48 degree 3 poles (-32.866, 8.3384) (-32.5507, 8.5085) (-32.2267, 8.5936) (-31.8926, 8.5936) knots 0 0 0 0 1 1 1 1
  spline S49 degree 3 poles (-31.8926, 8.5936) (-31.5623, 8.5936) (-31.2408, 8.5085) (-30.9267, 8.3384) knots 0 0 0 0 1 1 1 1
  spline S50 degree 3 poles (-30.9267, 8.3384) (-30.6115, 8.1682) (-30.365, 7.9242) (-30.1861, 7.6077) knots 0 0 0 0 1 1 1 1
  spline S51 degree 3 poles (-30.1861, 7.6077) (-30.0078, 7.2924) (-29.9183, 6.9634) (-29.9183, 6.6218) knots 0 0 0 0 1 1 1 1
  spline S52 degree 3 poles (-29.9183, 6.6218) (-29.9183, 6.2796) (-30.0053, 5.9518) (-30.1786, 5.6384) knots 0 0 0 0 1 1 1 1
  spline S53 degree 3 poles (-30.1786, 5.6384) (-30.3525, 5.3263) (-30.5958, 5.0835) (-30.9092, 4.9103) knots 0 0 0 0 1 1 1 1
  spline S54 degree 3 poles (-30.9092, 4.9103) (-31.2233, 4.7363) (-31.5511, 4.65) (-31.8926, 4.65) knots 0 0 0 0 1 1 1 1
  spline S55 degree 3 poles (-31.8926, 4.65) (-32.2329, 4.65) (-32.5601, 4.7363) (-32.8735, 4.9103) knots 0 0 0 0 1 1 1 1
  spline S56 degree 3 poles (-32.8735, 4.9103) (-33.1875, 5.0835) (-33.4309, 5.3263) (-33.6042, 5.6384) knots 0 0 0 0 1 1 1 1
  spline S57 degree 3 poles (-33.6042, 5.6384) (-33.7781, 5.9518) (-33.8644, 6.2796) (-33.8644, 6.6218) knots 0 0 0 0 1 1 1 1
  spline S58 degree 3 poles (-40.8214, 4.8952) (-40.8652, 4.8164) (-40.9265, 4.7564) (-41.0066, 4.7151) knots 0 0 0 0 1 1 1 1
  spline S59 degree 3 poles (-41.0066, 4.7151) (-41.0854, 4.6732) (-41.1654, 4.6525) (-41.2468, 4.6525) knots 0 0 0 0 1 1 1 1
  line L16 (-41.2468, 4.6525) -> (-44.1994, 4.6525)
  spline S60 degree 3 poles (-44.1994, 4.6525) (-44.2833, 4.6525) (-44.364, 4.6732) (-44.4422, 4.7151) knots 0 0 0 0 1 1 1 1
  spline S61 degree 3 poles (-44.4422, 4.7151) (-44.521, 4.7564) (-44.5823, 4.8164) (-44.6273, 4.8952) knots 0 0 0 0 1 1 1 1
  spline S62 degree 3 poles (-44.6273, 4.8952) (-44.6711, 4.9753) (-44.6924, 5.0585) (-44.6924, 5.1455) knots 0 0 0 0 1 1 1 1
  spline S63 degree 3 poles (-44.6924, 5.1455) (-44.6924, 5.2305) (-44.4472, 5.766) (-43.9567, 6.7519) knots 0 0 0 0 1 1 1 1
  spline S64 degree 3 poles (-43.9567, 6.7519) (-43.465, 7.7391) (-43.1979, 8.272) (-43.156, 8.3509) knots 0 0 0 0 1 1 1 1
  spline S65 degree 3 poles (-43.156, 8.3509) (-43.1128, 8.4291) (-43.0522, 8.4897) (-42.9733, 8.5335) knots 0 0 0 0 1 1 1 1
  spline S66 degree 3 poles (-42.9733, 8.5335) (-42.8951, 8.5767) (-42.8126, 8.5986) (-42.7256, 8.5986) knots 0 0 0 0 1 1 1 1
  spline S67 degree 3 poles (-42.7256, 8.5986) (-42.6405, 8.5986) (-42.5598, 8.5767) (-42.4829, 8.5335) knots 0 0 0 0 1 1 1 1
  spline S68 degree 3 poles (-42.4829, 8.5335) (-42.4047, 8.4897) (-42.344, 8.4291) (-42.3002, 8.3509) knots 0 0 0 0 1 1 1 1
  spline S69 degree 3 poles (-42.3002, 8.3509) (-42.2571, 8.272) (-41.9887, 7.7391) (-41.4945, 6.7519) knots 0 0 0 0 1 1 1 1
  spline S70 degree 3 poles (-41.4945, 6.7519) (-41.0009, 5.766) (-40.7538, 5.2305) (-40.7538, 5.1455) knots 0 0 0 0 1 1 1 1
  spline S71 degree 3 poles (-40.7538, 5.1455) (-40.7538, 5.0585) (-40.7763, 4.9753) (-40.8214, 4.8952) knots 0 0 0 0 1 1 1 1
  spline S72 degree 3 poles (-56.0227, 4.655) (-56.3498, 4.655) (-56.5144, 4.8139) (-56.5156, 5.133) knots 0 0 0 0 1 1 1 1
  line L17 (-56.5156, 5.133) -> (-56.5156, 8.1006)
  spline S73 degree 3 poles (-56.5156, 8.1006) (-56.5144, 8.4259) (-56.3498, 8.5917) (-56.0227, 8.5986) knots 0 0 0 0 1 1 1 1
  line L18 (-56.0227, 8.5986) -> (-53.5304, 8.5936)
  spline S74 degree 3 poles (-53.5304, 8.5936) (-53.2239, 8.5886) (-53.0694, 8.4291) (-53.0675, 8.1157) knots 0 0 0 0 1 1 1 1
  spline S75 degree 3 poles (-53.0675, 8.1157) (-53.0675, 7.7804) (-53.2339, 7.6102) (-53.5654, 7.6052) knots 0 0 0 0 1 1 1 1
  line L19 (-53.5654, 7.6052) -> (-55.5272, 7.6052)
  line L20 (-55.5272, 7.6052) -> (-55.5272, 5.6434)
  line L21 (-55.5272, 5.6434) -> (-53.5704, 5.6434)
  spline S76 degree 3 poles (-53.5704, 5.6434) (-53.2389, 5.6415) (-53.0725, 5.4758) (-53.0725, 5.1455) knots 0 0 0 0 1 1 1 1
  spline S77 degree 3 poles (-53.0725, 5.1455) (-53.0744, 4.8214) (-53.237, 4.6582) (-53.5604, 4.655) knots 0 0 0 0 1 1 1 1
  line L22 (-53.5604, 4.655) -> (-56.0227, 4.655)
  spline S78 degree 3 poles (-59.9613, 4.655) (-60.2884, 4.655) (-60.4529, 4.8139) (-60.4542, 5.133) knots 0 0 0 0 1 1 1 1
  line L23 (-60.4542, 5.133) -> (-60.4542, 8.1006)
  spline S79 degree 3 poles (-60.4542, 8.1006) (-60.4529, 8.4259) (-60.2884, 8.5917) (-59.9613, 8.5986) knots 0 0 0 0 1 1 1 1
  spline S80 degree 3 poles (-59.9613, 8.5986) (-59.631, 8.5898) (-59.4646, 8.4291) (-59.4608, 8.1157) knots 0 0 0 0 1 1 1 1
  line L24 (-59.4608, 8.1157) -> (-59.4658, 5.6434)
  line L25 (-59.4658, 5.6434) -> (-57.509, 5.6434)
  spline S81 degree 3 poles (-57.509, 5.6434) (-57.1775, 5.6415) (-57.0111, 5.4758) (-57.0111, 5.1455) knots 0 0 0 0 1 1 1 1
  spline S82 degree 3 poles (-57.0111, 5.1455) (-57.013, 4.8214) (-57.1756, 4.6582) (-57.499, 4.655) knots 0 0 0 0 1 1 1 1
  line L26 (-57.499, 4.655) -> (-59.9613, 4.655)
  line L27 (-47.4024, 7.6052) -> (-48.1405, 7.6052)
  spline S83 degree 3 poles (-48.1405, 7.6052) (-48.4696, 7.6052) (-48.6335, 7.7703) (-48.6335, 8.1006) knots 0 0 0 0 1 1 1 1
  spline S84 degree 3 poles (-48.6335, 8.1006) (-48.6322, 8.4259) (-48.4677, 8.5917) (-48.1405, 8.5986) knots 0 0 0 0 1 1 1 1
  line L28 (-48.1405, 8.5986) -> (-45.6483, 8.5936)
  spline S85 degree 3 poles (-45.6483, 8.5936) (-45.3418, 8.5886) (-45.1872, 8.4291) (-45.1854, 8.1157) knots 0 0 0 0 1 1 1 1
  spline S86 degree 3 poles (-45.1854, 8.1157) (-45.1854, 7.7804) (-45.3518, 7.6102) (-45.6833, 7.6052) knots 0 0 0 0 1 1 1 1
  line L29 (-45.6833, 7.6052) -> (-46.419, 7.6052)
  line L30 (-46.419, 7.6052) -> (-46.4165, 5.1455)
  spline S87 degree 3 poles (-46.4165, 5.1455) (-46.4202, 4.8214) (-46.5854, 4.6582) (-46.9119, 4.655) knots 0 0 0 0 1 1 1 1
  spline S88 degree 3 poles (-46.9119, 4.655) (-47.241, 4.655) (-47.4049, 4.8139) (-47.4049, 5.133) knots 0 0 0 0 1 1 1 1
  line L31 (-47.4049, 5.133) -> (-47.4024, 7.6052)
  spline S89 degree 3 poles (-24.9921, 6.6218) (-24.9921, 6.9634) (-24.9045, 7.2924) (-24.7293, 7.6077) knots 0 0 0 0 1 1 1 1
  spline S90 degree 3 poles (-24.7293, 7.6077) (-24.5529, 7.9242) (-24.3077, 8.1682) (-23.9937, 8.3384) knots 0 0 0 0 1 1 1 1
  spline S91 degree 3 poles (-23.9937, 8.3384) (-23.6784, 8.5085) (-23.3544, 8.5936) (-23.0203, 8.5936) knots 0 0 0 0 1 1 1 1
  spline S92 degree 3 poles (-23.0203, 8.5936) (-22.69, 8.5936) (-22.3685, 8.5085) (-22.0544, 8.3384) knots 0 0 0 0 1 1 1 1
  spline S93 degree 3 poles (-22.0544, 8.3384) (-21.7391, 8.1682) (-21.4927, 7.9242) (-21.3138, 7.6077) knots 0 0 0 0 1 1 1 1
  spline S94 degree 3 poles (-21.3138, 7.6077) (-21.1355, 7.2924) (-21.046, 6.9634) (-21.046, 6.6218) knots 0 0 0 0 1 1 1 1
  spline S95 degree 3 poles (-21.046, 6.6218) (-21.046, 6.2796) (-21.133, 5.9518) (-21.3063, 5.6384) knots 0 0 0 0 1 1 1 1
  spline S96 degree 3 poles (-21.3063, 5.6384) (-21.4802, 5.3263) (-21.7235, 5.0835) (-22.0369, 4.9103) knots 0 0 0 0 1 1 1 1
  spline S97 degree 3 poles (-22.0369, 4.9103) (-22.3509, 4.7363) (-22.6787, 4.65) (-23.0203, 4.65) knots 0 0 0 0 1 1 1 1
  spline S98 degree 3 poles (-23.0203, 4.65) (-23.3606, 4.65) (-23.6878, 4.7363) (-24.0012, 4.9103) knots 0 0 0 0 1 1 1 1
  spline S99 degree 3 poles (-24.0012, 4.9103) (-24.3152, 5.0835) (-24.5586, 5.3263) (-24.7319, 5.6384) knots 0 0 0 0 1 1 1 1
  spline S100 degree 3 poles (-24.7319, 5.6384) (-24.9058, 5.9518) (-24.9921, 6.2796) (-24.9921, 6.6218) knots 0 0 0 0 1 1 1 1
  arc A0 (-62.7452, 16.4403) -> (-67.7452, 11.4403) centre (-62.7452, 11.4403) ccw
  line L32 (-67.7452, 11.4403) -> (-67.7452, 1.4403)
  arc A1 (-67.7452, 1.4403) -> (-62.7452, -3.5597) centre (-62.7452, 1.4403) ccw
  line L33 (-62.7452, -3.5597) -> (-22.7452, -3.5597)
  arc A2 (-22.7452, -3.5597) -> (-17.7452, 1.4403) centre (-22.7452, 1.4403) ccw
  line L34 (-17.7452, 1.4403) -> (-17.7452, 11.4403)
  arc A3 (-17.7452, 11.4403) -> (-22.7452, 16.4403) centre (-22.7452, 11.4403) ccw
  line L35 (-22.7452, 16.4403) -> (-62.7452, 16.4403)
